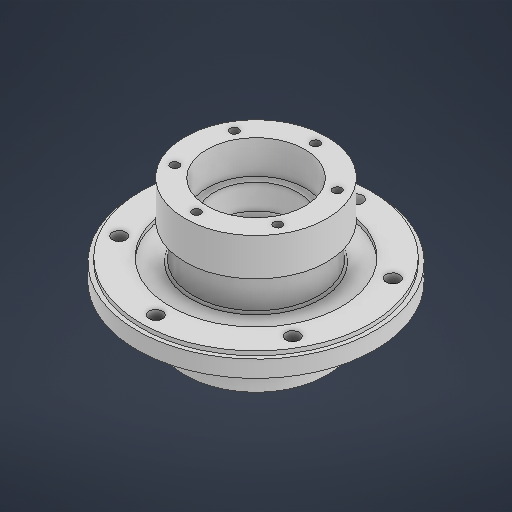
# Autodesk Inventor part: 11
Saved by Autodesk Inventor 2026.2 (Build 302298010, 298A)
## iProperties
Created: 2026-03-11
Part Number: 11
Material: Generico
Document SubType Name: Modeling
Designer: mahsa
Density: 1 g/cm^3
Appearance: Default
Author: mahsa
Autodesk Inventor part; units mm, degrees
ref_plane "YZ Plane" through (0, 0, 0) normal (1, 0, 0) x (0, 1, 0)
ref_plane "XZ Plane" through (0, 0, 0) normal (0, 1, 0) x (-1, 0, 0)
ref_plane "XY Plane" through (0, 0, 0) normal (0, 0, 1) x (1, 0, 0)
sketch "Schizzo1" plane through (0, 0, 0) normal (1, 0, 0) x (0, 1, 0)
  line L0 (870.2101, 0) -> (33.7001, 0)
  line L1 (838.8366, -23.5) -> (838.8366, -34)
  line L2 (838.8366, -34) -> (820.8366, -34)
  line L3 (838.8366, -23.5) -> (822.8366, -23.5)
  line L4 (822.8366, -23.5) -> (822.8366, -20)
  line L5 (822.8366, -20) -> (810.8366, -20)
  line L6 (810.8366, -20) -> (810.8366, -16)
  line L7 (801.8366, -16) -> (801.8366, -20)
  line L8 (801.8366, -20) -> (789.8366, -20)
  line L9 (789.8366, -20) -> (789.8366, -23.5)
  line L10 (789.8366, -23.5) -> (773.8366, -23.5)
  line L11 (773.8366, -23.5) -> (773.8366, -34)
  line L12 (773.8366, -34) -> (788.8366, -34)
  line L13 (788.8366, -34) -> (788.8366, -36)
  line L14 (788.8366, -36) -> (795.8366, -36)
  line L15 (820.8366, -34) -> (820.8366, -30)
  line L16 (795.8366, -36) -> (795.8366, -48)
  line L17 (805.8366, -48) -> (805.8366, -44.75)
  line L18 (805.8366, -44.75) -> (795.8366, -44.75)
  line L19 (805.8366, -41) -> (805.8366, -55)
  line L20 (795.8366, -48) -> (795.8366, -51.25)
  line L21 (795.8366, -51.25) -> (805.8366, -51.25)
  line L22 (805.8366, -55) -> (803.8366, -55)
  line L23 (803.8366, -55) -> (803.8366, -57)
  line L24 (803.8366, -57) -> (795.8366, -57)
  line L25 (795.8366, -57) -> (795.8366, -51.25)
  line L26 (805.8366, -41) -> (803.8366, -41)
  line L27 (803.8366, -41) -> (803.8366, -30)
  line L28 (810.8366, -16) -> (801.8366, -16)
  line L29 (820.8366, -30) -> (803.8366, -30)
  point P0 (0, 0)
  dimension "d1" = 10.5
  dimension "d2" = 18
  dimension "d3" = 16
  dimension "d4" = 3.5
  dimension "d5" = 12
  dimension "d6" = 4
  dimension "d8" = 4
  dimension "d9" = 12
  dimension "d10" = 3.5
  dimension "d11" = 16
  dimension "d12" = 15
  dimension "d13" = 2
  dimension "d14" = 7
  dimension "d23" = 4
  dimension "d25" = 12
  dimension "d26" = 10
  dimension "d29" = 3.25
  dimension "d30" = 14
  dimension "d31" = 3.25
  dimension "d32" = 10
  dimension "d33" = 2
  dimension "d34" = 2
  dimension "d35" = 8
  dimension "d36" = 2
  dimension "d37" = 9
  constraints: 60 end point, 12 perpendicular, 6 point on line, 6 vertical, 5 horizontal, 1 midpoint
  measures "d1" distance of L1.start L1.end
  measures "d2" distance of L1.end L2.end
  measures "d3" distance of L1.start L3.end
  measures "d4" distance of L3.end L4.end
  measures "d5" distance of L4.end L5.end
  measures "d6" distance of L5.end L6.end
  measures "d8" distance of L7.start L7.end
  measures "d9" distance of L7.end L8.end
  measures "d10" distance of L8.end L9.end
  measures "d11" distance of L9.end L10.end
  measures "d12" distance of L11.end L12.end
  measures "d13" distance of L12.end L13.end
  measures "d14" distance of L13.end L14.end
  measures "d23" distance of L2.end L15.end
  measures "d25" distance of L14.end L16.end
  measures "d26" distance of L16.end L17.start
  measures "d29" distance of L17.start L17.end
  measures "d30" distance of L19.start L19.end
  measures "d31" distance of L16.end L20.end
  measures "d32" distance of L20.end L21.end
  measures "d33" distance of L19.end L22.end
  measures "d34" distance of L22.end L23.end
  measures "d35" distance of L23.end L24.end
  measures "d36" distance of L19.start L26.end
  measures "d37" distance of L6.end L7.start
revolve "Rivoluzione1" add sketch "Schizzo1" angle 360 about axis through (0, 870.2101, 0) along (0, -1, 0)
sketch "Schizzo2" plane through (0, 805.8366, 0) normal (0, 1, 0) x (1, 0, 0)
  point P0 (0, 0)
sketch "Schizzo3" plane through (0, 805.8366, 0) normal (0, 1, 0) x (1, 0, 0)
  circle A0 centre (0, 0) radius 48
  circle A1 centre (0, 48) radius 3.25
  circle A2 centre (-41.5692, 24) radius 3.25
  circle A3 centre (-41.5692, -24) radius 3.25
  circle A4 centre (0, -48) radius 3.25
  circle A5 centre (41.5692, -24) radius 3.25
  circle A6 centre (41.5692, 24) radius 3.25
  dimension "d39" = 96
  dimension "d40" = 6.5
  dimension "d43" = 360
  constraints: 7 coincident, 6 centre point, 1 vertical alignment, 21 other
  measures "d40" diameter of A1
extrude "Estrusione1" cut sketch "Schizzo3" against normal up to next contours A6 A0 | A0 A6 | A5 A0 | A0 A5 | A1 A0 | A0 A1 | A4 A0 | A0 A4 | A2 A0 | A0 A2 | A3 A0 | A0 A3
sketch "Schizzo4" plane through (0, 773.8366, 0) normal (0, -1, 0) x (1, 0, 0)
  circle A0 centre (0, 0) radius 29
  point P0 (0, 29)
  point P1 (-25.1147, 14.5)
  point P2 (-25.1147, -14.5)
  point P3 (0, -29)
  point P4 (25.1147, -14.5)
  point P5 (25.1147, 14.5)
  dimension "d47" = 58
  dimension "d50" = 360
  constraints: 1 coincident, 1 vertical alignment, 9 other
hole "Foro1" at (0, 773.8366, 29) at (-25.1147, 773.8366, 14.5) at (-25.1147, 773.8366, -14.5) at (0, 773.8366, -29) at (25.1147, 773.8366, -14.5) at (25.1147, 773.8366, 14.5) direction (0, 1, 0) diameter 4.134 depth 14.6 tip angle 118 thread size "M5x0.8" class "6H" standard "ISO Metric profile"
sketch "Schizzo5" plane through (0, 838.8366, 0) normal (0, 1, 0) x (1, 0, 0)
  circle A0 centre (0, 0) radius 16 projected
  circle A1 centre (0, 0) radius 28.5
  point P0 (0, 28.5)
  point P1 (-24.6817, 14.25)
  point P2 (-24.6817, -14.25)
  point P3 (0, -28.5)
  point P4 (24.6817, -14.25)
  point P5 (24.6817, 14.25)
  dimension "d59" = 57
  dimension "d62" = 360
  constraints: 1 coincident, 1 vertical alignment, 9 other
hole "Foro2" at (0, 838.8366, -28.5) at (-24.6817, 838.8366, -14.25) at (-24.6817, 838.8366, 14.25) at (0, 838.8366, 28.5) at (24.6817, 838.8366, 14.25) at (24.6817, 838.8366, -14.25) direction (0, -1, 0) diameter 4.134 depth 14 tip angle 118 thread size "M5x0.8" class "6H" standard "ISO Metric profile"
fillet "Raccordo1" radius 1 1 edges at (0, 795.8366, 36) inverted yes
fillet "Raccordo2" radius 1 1 edges at (0, 803.8366, 30) inverted yes
